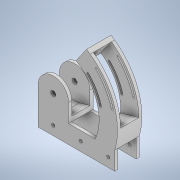
# Autodesk Inventor part: force_measurement_plate
Saved by Autodesk Inventor 2022 (Build 260153000, 153)
## iProperties
Created: 2022-01-31
Part Number: force_measurement_plate
Material: Generic
Document SubType Name: Modeling
Designer: Martijn
Density: 1 g/cm^3
Appearance: Default
Author: Martijn
Autodesk Inventor part; units mm, degrees
ref_plane "YZ Plane" through (0, 0, 0) normal (1, 0, 0) x (0, 1, 0)
ref_plane "XZ Plane" through (0, 0, 0) normal (0, 1, 0) x (-1, 0, 0)
ref_plane "XY Plane" through (0, 0, 0) normal (0, 0, 1) x (1, 0, 0)
sketch "Sketch1" plane through (0, 0, 0) normal (0, 0, 1) x (1, 0, 0)
  line L0 (0, 0) -> (0, 60)
  arc A0 (50, 60) -> (0, 60) centre (25, 60) ccw
  line L1 (50, 60) -> (50, 30)
  line L2 (50, 30) -> (93.7386, 30)
  line L3 (125.6231, 30) -> (125.6231, 0)
  line L4 (125.6231, 0) -> (0, 0)
  circle A1 centre (25, 60) radius 4.1
  arc A2 (93.7386, 30) -> (68.0182, 121.4364) centre (25, 60) ccw
  arc A3 (125.6231, 30) -> (85.2255, 146.011) centre (25, 60) ccw
  line L5 (68.0182, 121.4364) -> (85.2255, 146.011)
  line L6 (68.0182, 121.4364) -> (25, 60)
  dimension "d0" = 30
  dimension "d1" = 50
  dimension "d2" = 8.2
  dimension "d3" = 30
  dimension "d30" = 55
  dimension "d32" = 30
  dimension "d33" = 75
  dimension "d34" = 105
  constraints: 14 end point, 6 point on circle, 4 centre point, 3 coincident, 2 perpendicular, 2 tangent, 2 vertical, 1 collinear
  measures "d0" distance between parallel lines of L4 L2
  measures "d1" distance between parallel lines of L0 L1
  measures "d2" diameter of A1
  measures "d3" distance of L1.end L1.start
  measures "d30" angle of L2 L6
  measures "d32" distance of L3.start L3.end
  measures "d33" radius of A2
  measures "d34" distance of A0.centre L5.end
extrude "Extrusion1" add sketch "Sketch1" along normal blind 5 contours L0 A0 L1 L2 A2 L5 A3 L3 L4
sketch "Sketch2" plane through (0, 0, 5) normal (0, 0, 1) x (1, 0, 0)
  circle A0 centre (25, 15) radius 2.5
  line L0 (0, 0) -> (125.6231, 0) projected
  line L1 (0, 60) -> (0, 0) projected
  dimension "d18" = 15
  dimension "d19" = 25
  dimension "d20" = 5
  constraints: 1 centre point
  measures "d18" distance from line of L0 A0.centre
  measures "d19" distance from line of L1 A0.centre
  measures "d20" diameter of A0
extrude "Extrusion2" cut sketch "Sketch2" against normal blind 10
pattern_linear "Rectangular Pattern1" count 3 spacing 45 along (1, 0, 0) of "Extrusion2"
sketch "Sketch4" plane through (0, 0, 5) normal (0, 0, 1) x (1, 0, 0)
  circle A0 centre (25, 60) radius 4.1 projected
  line L0 (0, 60) -> (0, 0) projected
  arc A1 (0, 47.3905) -> (32.7178, 33.0847) centre (25, 60) ccw
  line L1 (32.7178, 33.0847) -> (50, 38.0403)
  line L2 (50, 30) -> (50, 60) projected
  line L3 (0, 47.3905) -> (0, 30)
  line L4 (93.7386, 30) -> (50, 30) projected
  line L5 (0, 30) -> (50, 30)
  line L6 (50, 30) -> (50, 38.0403)
  dimension "d26" = 28
  dimension "d27" = 16
  constraints: 8 end point, 2 point on circle, 2 point on line, 1 centre point, 1 coincident, 1 horizontal, 1 midpoint, 1 perpendicular, 1 tangent
  measures "d26" radius of A1
  measures "d27" angle of L5 L1
extrude "Extrusion3" add sketch "Sketch4" along normal blind 15 contours A1 L1 L2 L5 L0
sketch "Sketch5" plane through (0, 0, 5) normal (0, 0, 1) x (1, 0, 0)
  circle A0 centre (25, 60) radius 4.1 projected
  arc A1 (100.7286, 80.2914) -> (80.4372, 115.4372) centre (25, 60) ccw
  arc A2 (103.8195, 81.1196) -> (82.6999, 117.6999) centre (25, 60) ccw
  arc A3 (120.0471, 85.4678) -> (94.5793, 129.5793) centre (25, 60) ccw
  arc A4 (123.1381, 86.296) -> (96.842, 131.842) centre (25, 60) ccw
  arc A5 (82.6999, 117.6999) -> (80.4372, 115.4372) centre (81.5685, 116.5685) ccw
  arc A6 (100.7286, 80.2914) -> (103.8195, 81.1196) centre (102.2741, 80.7055) ccw
  arc A7 (96.842, 131.842) -> (94.5793, 129.5793) centre (95.7107, 130.7107) ccw
  arc A8 (120.0471, 85.4678) -> (123.1381, 86.296) centre (121.5926, 85.8819) ccw
  line L0 (95.7107, 130.7107) -> (81.5685, 116.5685)
  line L1 (81.5685, 116.5685) -> (25, 60)
  line L2 (25, 60) -> (102.2741, 80.7055)
  line L3 (102.2741, 80.7055) -> (121.5926, 85.8819)
  line L4 (93.7386, 30) -> (50, 30) projected
  point P0 (0, 0)
  dimension "d35" = 3.2
  dimension "d36" = 3.2
  dimension "d37" = 45
  dimension "d38" = 15
  dimension "d44" = 80
  dimension "d45" = 20
  constraints: 16 point on circle, 8 centre point, 8 end point, 8 tangent, 4 coincident, 2 collinear
  measures "d35" radial gap between concentric circles of A1 A2
  measures "d36" radial gap between concentric circles of A3 A4
  measures "d37" angle of L4 L1
  measures "d38" angle of L4 L2
  measures "d44" distance of A1.centre L0.end
  measures "d45" distance of L0.end L0.start
extrude "Extrusion4" cut sketch "Sketch5" against normal blind 15 contours L2 L3 A6 | A1 L1 L0 A2 L3 L2 | A5 L0 L1 | A3 A7 A4 A8
sketch "Sketch6" plane through (0, 0, 5) normal (0, 0, 1) x (1, 0, 0)
  circle A0 centre (25, 60) radius 4.1 projected
  arc A1 (125.6231, 30) -> (85.2255, 146.011) centre (25, 60) ccw projected
  arc A2 (125.6231, 30) -> (129.9954, 60.9786) centre (25, 60) ccw
  arc A3 (93.7386, 30) -> (68.0182, 121.4364) centre (25, 60) ccw projected
  arc A4 (93.7386, 30) -> (99.5998, 52.2628) centre (25, 60) ccw
  line L0 (99.5998, 52.2628) -> (129.9954, 60.9786)
  line L1 (93.7386, 30) -> (125.6231, 30)
  line L2 (50, 38.0403) -> (32.7178, 33.0847) projected
  point P0 (0, 0)
  constraints: 6 point on circle, 4 end point, 2 centre point, 2 coincident, 1 collinear, 1 horizontal
extrude "Extrusion5" add sketch "Sketch6" along normal blind 15 contours L1 A3 L0 A1
mirror "Mirror1" about plane through (111.8693, 45.4893, 20) normal (0, 0, 1)
sketch "Sketch7" plane through (68.0182, 121.4364, 0) normal (-0.8192, 0.5736, 0) x (0, 0, 1)
  line L0 (0, -41.8595) -> (0, 30) projected
  line L1 (40, 30) -> (35, 30) projected
  line L2 (0, 0) -> (40, 0)
  line L3 (40, 0) -> (40, 30)
  line L4 (40, 30) -> (0, 30)
  line L5 (0, 30) -> (0, 0)
  point P0 (0, -138.4885)
  point P1 (35, 30)
  point P2 (0, 30)
  constraints: 8 end point, 2 parallel, 1 collinear, 1 horizontal, 1 perpendicular
extrude "Extrusion6" add sketch "Sketch7" along normal blind 7
body "Solid1"
